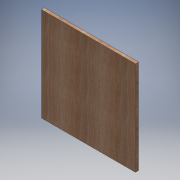
# Autodesk Inventor part: base
Saved by Autodesk Inventor 2019 (Build 230136000, 136)
## iProperties
Created: 2019-01-12
Part Number: base
Material: Wood (Birch)
Document SubType Name: Modeling
Designer: gaincarlo
Density: 0.55 g/cm^3
Appearance: Birch - Natural Polished
Project: La Panca - Flower Vase
Author: gaincarlo
Autodesk Inventor part; units mm, degrees
ref_plane "YZ Plane" through (0, 0, 0) normal (1, 0, 0) x (0, 1, 0)
ref_plane "XZ Plane" through (0, 0, 0) normal (0, 1, 0) x (-1, 0, 0)
ref_plane "Work Plane1" through (-33.0341, -79.7515, 0) normal (0, 0, 1) x (1, 0, 0)
sketch "Sketch1" plane through (-33.0341, -79.7515, 0) normal (0, 0, 1) x (1, 0, 0)
  line L0 (56.599, -392.8235) -> (56.599, -157.4952) construction
  line L1 (23.5648, -107.9033) -> (23.5648, 127.425) construction
  line L2 (56.599, -392.8235) -> (-543.401, -392.8235)
  line L3 (-543.401, -392.8235) -> (-543.401, 207.1765)
  line L4 (-543.401, 207.1765) -> (56.599, 207.1765)
  line L5 (56.599, 207.1765) -> (56.599, -392.8235)
  point P0 (33.0341, 79.7515)
  dimension "d0" = 600
  dimension "d1" = 600
  constraints: 8 end point, 2 parallel, 1 horizontal, 1 perpendicular
  measures "d0" distance of L3.end L4.end
  measures "d1" distance of L2.end L3.end
extrude "Extrusion1" add sketch "Sketch1" along normal blind 20
body "Solid1"
